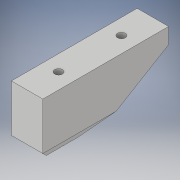
# Autodesk Inventor part: Slider
Saved by Autodesk Inventor 2019 (Build 230136000, 136)
## iProperties
Created: 2019-09-28
Part Number: Slider
Material: Generic
Document SubType Name: Modeling
Designer: james
Density: 1 g/cm^3
Appearance: Default
Author: james
Autodesk Inventor part; units mm, degrees
ref_plane "YZ Plane" through (0, 0, 0) normal (1, 0, 0) x (0, 1, 0)
ref_plane "XZ Plane" through (0, 0, 0) normal (0, 1, 0) x (-1, 0, 0)
ref_plane "XY Plane" through (0, 0, 0) normal (0, 0, 1) x (1, 0, 0)
sketch "Sketch1" plane through (0, 0, 0) normal (0, 0, 1) x (1, 0, 0)
  line L0 (-12.552, 15.5925) -> (0.148, 15.5925)
  line L1 (0.148, 15.5925) -> (0.148, -9.8075)
  line L2 (0.148, -9.8075) -> (-12.552, -9.8075)
  line L3 (-12.552, -9.8075) -> (-12.552, 15.5925)
  point P0 (0, 0)
  dimension "d0" = 12.7
  dimension "d1" = 25.4
  constraints: 8 end point, 2 parallel, 1 horizontal, 1 perpendicular
  measures "d0" distance of L1.end L2.end
  measures "d1" distance of L2.end L0.start
extrude "Extrusion1" add sketch "Sketch1" along normal blind 50.8
sketch "Sketch2" plane through (-12.552, 15.5925, 0) normal (0, 1, 0) x (1, 0, 0)
  line L0 (12.7, -50.8) -> (0, -50.8) projected
  line L1 (12.7, 0) -> (12.7, -50.8) projected
  point P0 (12.552, 0)
  point P1 (6.35, -38.1)
  point P2 (6.35, -12.7)
  dimension "d4" = 25.4
  dimension "d5" = 12.7
  dimension "d6" = 0
  dimension "d7" = 6.35
  measures "d4" distance of point (6.35, -38.1) point (6.35, -12.7)
  measures "d5" distance from line of L0 point (6.35, -38.1)
  measures "d6" horizontal distance of point (6.35, -38.1) point (6.35, -12.7)
  measures "d7" distance from line of L1 point (6.35, -12.7)
hole "Hole1" at (-6.202, 15.5925, 38.1) at (-6.202, 15.5925, 12.7) direction (0, -1, 0) diameter 3.175 end through all
sketch "Sketch3" plane through (0.148, -9.8075, 0) normal (1, 0, 0) x (0, 0, -1)
  line L0 (0, 0) -> (-50.8, 0) projected
  line L1 (0, 25.4) -> (-50.8, 25.4) projected
  line L2 (-50.8, 25.4) -> (0, 25.4)
  line L3 (0, 19.05) -> (-31.75, 0)
  line L4 (-31.75, 0) -> (-44.45, 0)
  line L5 (0, 0) -> (-50.8, 0) projected
  line L6 (-44.45, 0) -> (-50.8, 6.35)
  line L7 (-50.8, 0) -> (-44.3921, -0.0579)
  line L8 (-31.75, 0) -> (0, 0)
  line L9 (0, 19.05) -> (0, 0)
  line L10 (-50.8, 25.4) -> (-50.8, 0) projected
  line L11 (-50.8, 6.35) -> (-50.8, 0)
  point P0 (0, 9.8075)
  dimension "d18" = 12.7
  dimension "d19" = 19.05
  dimension "d20" = 6.35
  constraints: 16 end point, 2 horizontal, 2 point on line, 1 vertical
  measures "d18" distance of L4.end L3.end
  measures "d19" distance of L6.end L1.end
  measures "d20" distance of L1.start L3.start
extrude "Extrusion2" cut sketch "Sketch3" against normal blind 50.8
sketch "Sketch4" plane through (0, 0, 50.8) normal (0, 0, 1) x (1, 0, 0)
  line L0 (0.148, -9.8075) -> (-12.552, -9.8075) projected
  line L1 (-12.552, -9.8075) -> (-12.552, -3.4575) projected
  line L2 (0.148, -3.4575) -> (0.148, -9.8075) projected
  line L3 (-12.552, -3.4575) -> (0.148, -3.4575) projected
  line L4 (-12.552, -9.8075) -> (0.148, -9.8075) projected
  line L5 (-7.98, -9.8075) -> (-12.552, -9.8075)
  line L6 (-12.552, -9.8075) -> (-12.552, -3.4575)
  line L7 (-7.98, -9.8075) -> (-12.552, -3.4575)
  line L8 (0.148, -9.8075) -> (-4.805, -9.8075)
  line L9 (-4.805, -9.8075) -> (0.148, -3.4575)
  line L10 (0.148, -9.8075) -> (0.148, 9.2425) projected
  line L11 (0.148, -3.4575) -> (0.148, -9.8075)
  point P0 (0, 0)
  dimension "d23" = 3.175
  dimension "d24" = 4.572
  dimension "d25" = 4.953
  constraints: 12 end point, 3 collinear, 2 point on line
  measures "d23" distance of L5.start L8.end
  measures "d24" distance of L5.start L0.end
  measures "d25" distance of L0.start L8.end
extrude "Extrusion3" cut sketch "Sketch4" against normal blind 50.8 contours L0 L9 L2 | L0 L1 L7
body "Solid1"
